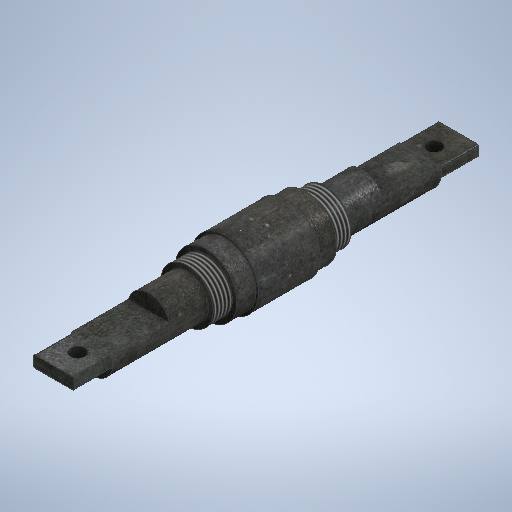
# Autodesk Inventor part: Shaft
Saved by Autodesk Inventor 2025.2 (Build 292293000, 293)
## iProperties
Created: 2025-05-25
Part Number: Shaft
Material: Steel
Document SubType Name: Modeling
Designer: Moaz
Density: 7.85 g/cm^3
Appearance: Plate
Author: Moaz
Autodesk Inventor part; units mm, degrees
ref_plane "YZ Plane" through (0, 0, 0) normal (1, 0, 0) x (0, 1, 0)
ref_plane "XZ Plane" through (0, 0, 0) normal (0, 1, 0) x (-1, 0, 0)
sketch "Sketch1" plane through (0, 0, 0) normal (0, 0, 1) x (1, 0, 0)
  circle A0 centre (0, 0) radius 32.5
  dimension "d0" = 65
  constraints: 1 centre point, 1 coincident
  measures "d0" diameter of A0
extrude "Extrusion1" add sketch "Sketch1" along normal blind 105
sketch "Sketch2" plane through (0, 0, 105) normal (0, 0, 1) x (1, 0, 0)
  circle A0 centre (0, 0) radius 27.5
  dimension "d3" = 55
  constraints: 1 centre point, 1 coincident
  measures "d3" diameter of A0
extrude "Extrusion2" add sketch "Sketch2" along normal blind 20
sketch "Sketch3" plane through (0, 0, 125) normal (0, 0, 1) x (1, 0, 0)
  circle A0 centre (0, 0) radius 22.5
  dimension "d6" = 45
  constraints: 1 centre point, 1 coincident
  measures "d6" diameter of A0
extrude "Extrusion3" add sketch "Sketch3" along normal blind 100
ref_plane "Work Plane1" through (0, 0, 52.5) normal (0, 0, -1) x (-1, 0, 0)
mirror "Mirror1" about plane through (0, 0, 52.5) normal (0, 0, -1) of "Extrusion3", "Extrusion2"
sketch "Sketch7" plane through (0, 0, -120) normal (0, 0, -1) x (-1, 0, 0)
  point P0 (0, 0)
sketch "Sketch11" plane through (0, 0, 52.5) normal (0, 0, -1) x (-1, 0, 0)
  circle A0 centre (0, 0) radius 35
  dimension "d43" = 70
  constraints: 1 centre point, 1 coincident
  measures "d43" diameter of A0
extrude "Extrusion9" add sketch "Sketch11" along normal mid plane 65
sketch "Sketch12" plane through (0, 0, 225) normal (0, 0, 1) x (1, 0, 0)
  circle A0 centre (0, 0) radius 22.5 projected
  line L0 (-19.6852, 6) -> (19.6852, 6)
  line L1 (21.6852, 4) -> (21.6852, -4)
  line L2 (19.6852, -6) -> (-19.6852, -6)
  line L3 (-21.6852, -4) -> (-21.6852, 4)
  arc A1 (-19.6852, 6) -> (-21.6852, 4) centre (-19.6852, 4) ccw
  arc A2 (-21.6852, -4) -> (-19.6852, -6) centre (-19.6852, -4) ccw
  arc A3 (19.6852, -6) -> (21.6852, -4) centre (19.6852, -4) ccw
  arc A4 (21.6852, 4) -> (19.6852, 6) centre (19.6852, 4) ccw
  point P0 (-21.6852, 6)
  point P1 (21.6852, 6)
  point P2 (21.6852, -6)
  point P3 (-21.6852, -6)
  dimension "d47" = 12
  dimension "d48" = 2
  constraints: 12 point on circle, 8 end point, 8 point on line, 8 tangent, 4 centre point, 3 equal radius, 3 perpendicular, 1 horizontal
  measures "d47" distance between parallel lines of L2 L0
  measures "d48" radius of A1
extrude "Extrusion10" add sketch "Sketch12" along normal blind 30 contours L0 A4 L1 A3 L2 A2 L3 A1
sketch "Sketch13" plane through (-19.6852, 6, 225) normal (0, 1, 0) x (1, 0, 0)
  circle A0 centre (19.6852, -15) radius 7.5
  line L0 (39.3705, -30) -> (0, -30) projected
  line L1 (39.3705, 0) -> (39.3705, -30) projected
  point P0 (19.6852, 225)
  dimension "d51" = 15
  dimension "d52" = 15
  dimension "d53" = 19.6852
  constraints: 1 centre point
  measures "d51" diameter of A0
  measures "d52" distance from line of L0 A0.centre
  measures "d53" distance from line of L1 A0.centre
extrude "Extrusion11" cut sketch "Sketch13" against normal through all
mirror "Mirror3" about plane through (0, 0, 52.5) normal (0, 0, -1) of "Extrusion10", "Extrusion11"
thread "Thread5" size "M55x4" class "6g" standard "ANSI Metric M Profile" full length
sketch "Sketch14" plane through (0, 0, 225) normal (0, 0, 1) x (1, 0, 0)
  arc A0 (-21.6852, -4) -> (-19.6852, -6) centre (-19.6852, -4) ccw projected
  line L0 (-21.6852, -4) -> (-21.6852, 4) projected
  arc A1 (-19.6852, 6) -> (-21.6852, 4) centre (-19.6852, 4) ccw projected
  line L1 (-19.6852, 6) -> (19.6852, 6) projected
  arc A2 (21.6852, 4) -> (19.6852, 6) centre (19.6852, 4) ccw projected
  line L2 (21.6852, 4) -> (21.6852, -4) projected
  arc A3 (19.6852, -6) -> (21.6852, -4) centre (19.6852, -4) ccw projected
  line L3 (19.6852, -6) -> (-19.6852, -6) projected
  circle A4 centre (0, 0) radius 22.5 projected
  line L4 (-19.6852, -6) -> (19.6852, -6) projected
  line L5 (-19.6852, -6) -> (-21.6852, -6)
  line L6 (19.6852, -6) -> (21.6852, -6)
  constraints: 4 end point, 2 horizontal, 2 point on circle
extrude "Extrusion12" [suppressed]
sketch "Sketch15" plane through (0, 0, -120) normal (0, 0, -1) x (-1, 0, 0)
  arc A0 (19.6852, -6) -> (21.6852, -4) centre (19.6852, -4) ccw projected
  line L0 (19.6852, -6) -> (-19.6852, -6) projected
  arc A1 (-21.6852, -4) -> (-19.6852, -6) centre (-19.6852, -4) ccw projected
  line L1 (-21.6852, -4) -> (-21.6852, 4) projected
  arc A2 (-19.6852, 6) -> (-21.6852, 4) centre (-19.6852, 4) ccw projected
  line L2 (-19.6852, 6) -> (19.6852, 6) projected
  arc A3 (21.6852, 4) -> (19.6852, 6) centre (19.6852, 4) ccw projected
  line L3 (21.6852, 4) -> (21.6852, -4) projected
  circle A4 centre (0, 0) radius 22.5 projected
  line L4 (-19.6852, -6) -> (-21.6852, -6)
  line L5 (19.6852, -6) -> (21.6852, -6)
  constraints: 4 end point, 2 horizontal, 2 point on circle
extrude "Extrusion13" [suppressed]
sketch "Sketch16" plane through (0, 0, 255) normal (0, 0, 1) x (1, 0, 0)
  line L0 (-19.6852, -6) -> (19.6852, -6) projected
  arc A0 (19.6852, -6) -> (21.6852, -4) centre (19.6852, -4) ccw projected
  line L1 (21.6852, -4) -> (21.6852, 4) projected
  arc A1 (21.6852, 4) -> (19.6852, 6) centre (19.6852, 4) ccw projected
  line L2 (19.6852, 6) -> (-19.6852, 6) projected
  arc A2 (-19.6852, 6) -> (-21.6852, 4) centre (-19.6852, 4) ccw projected
  line L3 (-21.6852, 4) -> (-21.6852, -4) projected
  arc A3 (-21.6852, -4) -> (-19.6852, -6) centre (-19.6852, -4) ccw projected
  point P0 (0, 0)
extrude "Extrusion14" add sketch "Sketch16" along normal blind 10
sketch "Sketch17" plane through (19.6852, -6, -150) normal (0, 0, -1) x (-1, 0, 0)
  line L0 (39.3705, 0) -> (0, 0) projected
  arc A0 (39.3705, 0) -> (41.3705, 2) centre (39.3705, 2) ccw projected
  line L1 (41.3705, 10) -> (41.3705, 2) projected
  arc A1 (41.3705, 10) -> (39.3705, 12) centre (39.3705, 10) ccw projected
  line L2 (0, 12) -> (39.3705, 12) projected
  arc A2 (0, 12) -> (-2, 10) centre (0, 10) ccw projected
  line L3 (-2, 2) -> (-2, 10) projected
  arc A3 (-2, 2) -> (0, 0) centre (0, 2) ccw projected
  point P0 (19.6852, 6)
extrude "Extrusion15" add sketch "Sketch17" along normal blind 10
sketch "Sketch18" plane through (0, 0, 225) normal (0, 0, 1) x (1, 0, 0)
  arc A0 (-21.6852, -4) -> (-19.6852, -6) centre (-19.6852, -4) ccw projected
  line L0 (-21.6852, -4) -> (-21.6852, 4) projected
  arc A1 (-19.6852, 6) -> (-21.6852, 4) centre (-19.6852, 4) ccw projected
  line L1 (-19.6852, 6) -> (19.6852, 6) projected
  arc A2 (21.6852, 4) -> (19.6852, 6) centre (19.6852, 4) ccw projected
  line L2 (21.6852, 4) -> (21.6852, -4) projected
  arc A3 (19.6852, -6) -> (21.6852, -4) centre (19.6852, -4) ccw projected
  line L3 (19.6852, -6) -> (-19.6852, -6) projected
  circle A4 centre (0, 0) radius 22.5 projected
  line L4 (-19.6852, 6) -> (-21.6852, 6)
  line L5 (19.6852, 6) -> (21.6852, 6)
  constraints: 4 end point, 2 horizontal, 2 point on circle
extrude "Extrusion16" cut sketch "Sketch18" against normal blind 60 contours L4 A4 L5 L1
sketch "Sketch19" plane through (0, 0, -120) normal (0, 0, -1) x (-1, 0, 0)
  arc A0 (19.6852, -6) -> (21.6852, -4) centre (19.6852, -4) ccw projected
  line L0 (19.6852, -6) -> (-19.6852, -6) projected
  arc A1 (-21.6852, -4) -> (-19.6852, -6) centre (-19.6852, -4) ccw projected
  line L1 (-21.6852, -4) -> (-21.6852, 4) projected
  arc A2 (-19.6852, 6) -> (-21.6852, 4) centre (-19.6852, 4) ccw projected
  line L2 (-19.6852, 6) -> (19.6852, 6) projected
  arc A3 (21.6852, 4) -> (19.6852, 6) centre (19.6852, 4) ccw projected
  line L3 (21.6852, 4) -> (21.6852, -4) projected
  circle A4 centre (0, 0) radius 22.5 projected
  line L4 (-19.6852, 6) -> (-21.6852, 6)
  line L5 (19.6852, 6) -> (21.6852, 6)
  constraints: 4 end point, 2 horizontal, 2 point on circle
extrude "Extrusion17" cut sketch "Sketch19" against normal blind 60 contours L2 L4 A4 L5
body "Solid1"
